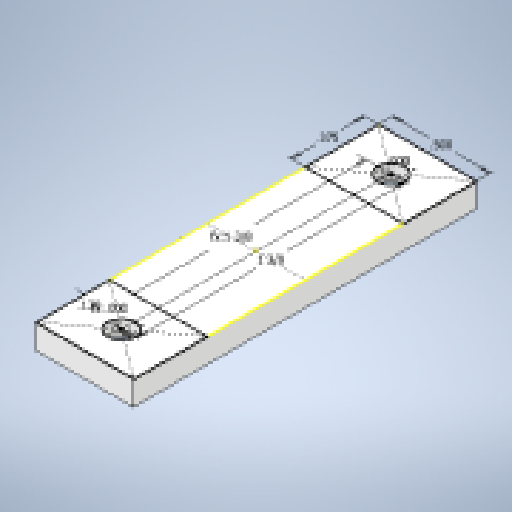
# Autodesk Inventor part: ramp
Saved by Autodesk Inventor 2023.2 (Build 272271000, 271)
## iProperties
Created: 2024-01-16
Part Number: ramp
Material: UHMW, White
Document SubType Name: Modeling
Designer: Nathan Cai
Mass: 1.25658 g
Surface Area: 14.8485 cm^2
Volume: 1.33679 cm^3
Density: 0.94 g/cm^3
Appearance: Smooth - White
Author: Nathan Cai
Autodesk Inventor part; units mm, degrees
ref_plane "YZ Plane" through (0, 0, 0) normal (1, 0, 0) x (0, 1, 0)
ref_plane "XZ Plane" through (0, 0, 0) normal (0, 1, 0) x (-1, 0, 0)
ref_plane "XY Plane" through (0, 0, 0) normal (0, 0, 1) x (1, 0, 0)
sketch "Sketch1" plane through (0, 0, 0) normal (0, 1, 0) x (-1, 0, 0)
  line L0 (-6.35, 22.225) -> (6.35, 22.225)
  line L1 (6.35, 22.225) -> (6.35, -22.225)
  line L2 (6.35, -22.225) -> (-6.35, -22.225)
  line L3 (-6.35, -22.225) -> (-6.35, 22.225)
  line L4 (-6.35, 22.225) -> (6.35, -22.225) construction
  line L5 (6.35, 22.225) -> (-6.35, -22.225) construction
  line L6 (-4.7625, 9.525) -> (4.7625, 9.525) construction
  line L7 (4.7625, 9.525) -> (4.7625, -9.525) construction
  line L8 (4.7625, -9.525) -> (-4.7625, -9.525) construction
  line L9 (-4.7625, -9.525) -> (-4.7625, 9.525) construction
  line L10 (-4.7625, 9.525) -> (4.7625, -9.525) construction
  line L11 (4.7625, 9.525) -> (-4.7625, -9.525) construction
  point P0 (0, 0)
  dimension "d0" = 12.7
  dimension "d1" = 44.45
  dimension "d2" = 9.525
  dimension "d3" = 19.05
  constraints: 24 end point, 4 midpoint, 4 parallel, 2 horizontal, 2 perpendicular
  measures "d0" distance of L1.end L2.end
  measures "d1" distance of L0.end L1.end
  measures "d2" distance of L7.end L8.end
  measures "d3" distance of L6.end L7.end
extrude "Extrusion1" add sketch "Sketch1" along normal blind 3.175
chamfer "Chamfer1" distance 3.175 distance2 6.35 1 edges at (-6.35, 0, 0) measured on face at (-6.35, 1.0583, -7.4083)
fillet "Fillet1" radius 3.175 1 edges at (-0.0005, 0, 0)
sketch "Sketch2" plane through (0, 3.175, 0) normal (0, 1, 0) x (1, 0, 0)
  line L0 (0, -17.4625) -> (0, -17.4625) construction
  line L1 (0, -17.4625) -> (0, 17.4625) construction
  line L2 (0, 17.4625) -> (0, 17.4625) construction
  line L3 (0, 17.4625) -> (0, -17.4625) construction
  line L4 (0, -17.4625) -> (0, 17.4625) construction
  line L5 (0, -17.4625) -> (0, 17.4625) construction
  circle A0 centre (0, -17.4625) radius 1.7526
  circle A1 centre (0, 17.4625) radius 1.7526
  circle A2 centre (0, -17.4625) radius 1.7526
  circle A3 centre (0, 17.4625) radius 1.7526
  line L6 (6.35, 12.7) -> (-6.35, 12.7)
  line L7 (-6.35, 12.7) -> (-6.35, 22.225)
  line L8 (-6.35, 22.225) -> (6.35, 22.225)
  line L9 (6.35, 22.225) -> (6.35, 12.7)
  line L10 (6.35, 12.7) -> (-6.35, 22.225) construction
  line L11 (-6.35, 12.7) -> (6.35, 22.225) construction
  line L12 (-6.35, 22.225) -> (-6.35, -22.225) projected
  line L13 (-6.35, 0) -> (6.35, 0) construction
  line L14 (6.35, -22.225) -> (6.35, 22.225) projected
  line L15 (6.35, -12.7) -> (-6.35, -12.7)
  line L16 (-6.35, -12.7) -> (-6.35, -22.225)
  line L17 (-6.35, -22.225) -> (6.35, -22.225)
  line L18 (6.35, -22.225) -> (6.35, -12.7)
  line L19 (6.35, -12.7) -> (-6.35, -22.225) construction
  line L20 (-6.35, -12.7) -> (6.35, -22.225) construction
  point P0 (0, 0)
  point P1 (0, 17.4625)
  point P2 (0, -17.4625)
  point P3 (0, -17.4625)
  point P4 (0, -17.4625)
  point P5 (6.35, -12.7)
  point P6 (-6.35, -12.7)
  point P7 (-6.35, -22.225)
  dimension "d10" = 0
  dimension "d11" = 34.925
  dimension "d12" = 3.5052
  dimension "d15" = 34.925
  dimension "d18" = 0
  dimension "d21" = 12.7
  dimension "d22" = 9.525
  constraints: 38 end point, 8 symmetric about line, 7 midpoint, 4 centre point, 4 equal length, 3 horizontal, 2 perpendicular, 1 coincident, 1 vertical, 5 other
  measures "d10" distance of L2.end L1.end
  measures "d11" distance of L1.end L0.end
  measures "d12" diameter of A0
  measures "d15" distance of A0.centre A1.centre
  measures "d18" distance of A0.centre A2.centre
  measures "d21" distance of L7.end L8.end
  measures "d22" distance of L6.end L7.end
extrude "Extrusion2" add sketch "Sketch2" against normal up to surface (3.175 mm away) contours A0 | A1 | L6 L7 L8 L9 | L14 L17 L12 L15
extrude "Extrusion3" cut sketch "Sketch2" against normal through all contours A0 | A1
chamfer "Chamfer2" distance 1.524 angle 49 2 edges at (-1.7526, 0, 17.4625) (-1.7526, 0, -17.4625) measured on face at (4.483, 0, 4.2333)
equation "\"d15\" = d11"
body "Solid1"
